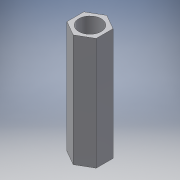
# Autodesk Inventor part: 15mmStandoff
Saved by Autodesk Inventor 2017 (Build 210142000, 142)
## iProperties
Created: 2019-06-27
Part Number: 15mmStandoff
Material: Generic
Document SubType Name: Modeling
Designer: cresswnd
Density: 1 g/cm^3
Appearance: White
Author: cresswnd
Autodesk Inventor part; units mm, degrees
ref_plane "YZ Plane" through (0, 0, 0) normal (1, 0, 0) x (0, 1, 0)
ref_plane "XZ Plane" through (0, 0, 0) normal (0, 1, 0) x (-1, 0, 0)
ref_plane "XY Plane" through (0, 0, 0) normal (0, 0, 1) x (1, 0, 0)
sketch "Sketch1" plane through (0, 0, 0) normal (0, 0, 1) x (1, 0, 0)
  circle A0 centre (0, 0) radius 2.25 construction
  circle A1 centre (0, 0) radius 1.5
  line L0 (0, 2.25) -> (1.9486, 1.125)
  line L1 (1.9486, 1.125) -> (1.9486, -1.125)
  line L2 (1.9486, -1.125) -> (0, -2.25)
  line L3 (0, -2.25) -> (-1.9486, -1.125)
  line L4 (-1.9486, -1.125) -> (-1.9486, 1.125)
  line L5 (-1.9486, 1.125) -> (0, 2.25)
  dimension "d0" = 4.5
  dimension "d1" = 3
  constraints: 12 end point, 3 coincident, 1 centre point, 1 vertical alignment, 15 other
  measures "d1" diameter of A1
extrude "Extrusion1" add sketch "Sketch1" along normal blind 15
body "Solid1"
